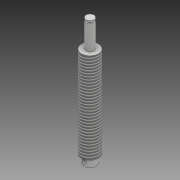
# Autodesk Inventor part: igus_6.35x2.54_screw
Saved by Autodesk Inventor 2017 SP1 (Build 210196100, 196)
## iProperties
Created: 2018-01-19
Part Number: igus_6.35x2.54_screw
Material: Generic
Document SubType Name: Modeling
Designer: Tomasz
Density: 1 g/cm^3
Appearance: Default
Author: Tomasz
Autodesk Inventor part; units mm, degrees
ref_plane "YZ Plane" through (0, 0, 0) normal (1, 0, 0) x (0, 1, 0)
ref_plane "XY Plane" through (0, 0, 0) normal (0, 0, 1) x (1, 0, 0)
sketch "Sketch1" plane through (0, 0, 0) normal (0, 1, 0) x (-1, 0, 0)
  line L0 (0, 9.9065) -> (0, -47)
  line L1 (0, -47) -> (2.25, -47)
  line L2 (2.25, -47) -> (2.25, -44)
  line L3 (2.25, -44) -> (3.175, -44)
  line L4 (3.175, -44) -> (3.175, -10.2)
  line L5 (3.175, -10.2) -> (1.5, -10.2)
  line L6 (1.5, -10.2) -> (1.5, -1)
  line L7 (1.5, -1) -> (1.1, -1)
  line L8 (1.1, -1) -> (1.1, -0.6)
  line L9 (1.1, -0.6) -> (1.5, -0.6)
  line L10 (1.5, -0.6) -> (1.5, 0)
  line L11 (1.5, 0) -> (0, 0)
  dimension "d0" = 33.8
  dimension "d1" = 3
  dimension "d2" = 10.2
  dimension "d3" = 4.5
  dimension "d4" = 6.35
  dimension "d5" = 3
  dimension "d6" = 0.4
  dimension "d7" = 2.2
  dimension "d29" = 1
  constraints: 26 end point, 7 perpendicular, 3 point on line, 1 horizontal, 1 vertical
  measures "d0" distance between parallel lines of L3 L5
  measures "d1" distance of L1.end L2.end
  measures "d2" distance between parallel lines of L5 L11
  measures "d3" diameter of L2 L0
  measures "d4" diameter of L4 L0
  measures "d5" diameter of L10 L0
  measures "d6" distance between parallel lines of L7 L9
  measures "d7" diameter of L8.end L0
  measures "d29" distance between parallel lines of L7 L11
revolve "Revolution1" add sketch "Sketch1" angle 360 about axis through (0, 0, 9.9065) along (0, 0, -1)
thread "Thread1" size "M7x1" class "6g" standard "ANSI Metric M Profile" full length
ref_plane "Work Plane1" through (0, 2.25, -45.5) normal (0, 1, 0) x (-1, 0, 0)
sketch "Sketch2" plane through (0, 2.25, -45.5) normal (0, 1, 0) x (-1, 0, 0)
  line L0 (-2.25, -1.5) -> (2.25, -1.5) projected
  line L1 (0, -1.5) -> (0, 45.5) construction
  point P0 (0, 0)
  dimension "d12" = 1.5
  constraints: 2 end point, 1 midpoint, 1 point on line, 1 vertical
  measures "d12" distance from line of point (0, 0) L0
hole "Hole1" at (0, 2.25, -45.5) direction (0, -1, 0) diameter 1.5 end through all
hole "Hole2" at (0, 0, -47) direction (0, 0, 1) diameter 3.1 depth 9 tip angle 118
body "Solid1"
